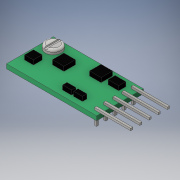
# Autodesk Inventor part: IMU
Saved by Autodesk Inventor 2016 (Build 200138000, 138)
## iProperties
Created: 2015-09-21
Part Number: IMU
Material: Generic
Document SubType Name: Modeling
Designer: lachesis
Density: 1 g/cm^3
Appearance: Default
Author: lachesis
Autodesk Inventor part; units mm, degrees
ref_plane "YZ Plane" through (0, 0, 0) normal (1, 0, 0) x (0, 1, 0)
ref_plane "XZ Plane" through (0, 0, 0) normal (0, 1, 0) x (-1, 0, 0)
ref_plane "XY Plane" through (0, 0, 0) normal (0, 0, 1) x (1, 0, 0)
sketch "Sketch1" plane through (0, 0, 0) normal (0, 1, 0) x (-1, 0, 0)
  line L0 (12.954, 6.731) -> (-12.954, 6.731)
  line L1 (-12.954, 6.731) -> (-12.954, -6.731)
  line L2 (-12.954, -6.731) -> (12.954, -6.731)
  line L3 (12.954, -6.731) -> (12.954, 6.731)
  point P0 (0, 0)
  point P1 (12.954, 0)
  point P2 (0, -6.731)
  dimension "d0" = 25.908
  dimension "d1" = 13.462
  constraints: 8 end point, 2 midpoint, 2 parallel, 1 horizontal, 1 horizontal alignment, 1 perpendicular, 1 vertical alignment
  measures "d0" distance of L1.end L2.end
  measures "d1" distance of L2.end L0.start
extrude "Extrusion1" add sketch "Sketch1" along normal blind 1.27
sketch "Sketch2" plane through (0, 1.27, 0) normal (0, 1, 0) x (1, 0, 0)
  circle A0 centre (-10.033, 3.81) radius 2.286
  line L0 (-12.954, 6.731) -> (-12.954, -6.731) projected
  line L1 (-11.303, -0.635) -> (-8.763, -0.635)
  line L2 (-8.763, -0.635) -> (-8.763, -3.175)
  line L3 (-8.763, -3.175) -> (-11.303, -3.175)
  line L4 (-11.303, -3.175) -> (-11.303, -0.635)
  line L5 (-12.954, -6.731) -> (12.954, -6.731) projected
  line L6 (-6.096, 2.921) -> (-2.794, 2.921)
  line L7 (-2.794, 2.921) -> (-2.794, -0.381)
  line L8 (-2.794, -0.381) -> (-6.096, -0.381)
  line L9 (-6.096, -0.381) -> (-6.096, 2.921)
  line L10 (12.954, 6.731) -> (-12.954, 6.731) projected
  line L11 (2.032, 5.461) -> (5.334, 5.461)
  line L12 (5.334, 5.461) -> (5.334, 2.159)
  line L13 (5.334, 2.159) -> (2.032, 2.159)
  line L14 (2.032, 2.159) -> (2.032, 5.461)
  line L15 (12.954, -6.731) -> (12.954, 6.731) projected
  line L16 (6.858, 4.699) -> (9.906, 4.699)
  line L17 (9.906, 4.699) -> (9.906, 2.667)
  line L18 (9.906, 2.667) -> (6.858, 2.667)
  line L19 (6.858, 2.667) -> (6.858, 4.699)
  line L20 (1.651, -3.937) -> (4.191, -3.937)
  line L21 (4.191, -3.937) -> (4.191, -5.207)
  line L22 (4.191, -5.207) -> (1.651, -5.207)
  line L23 (1.651, -5.207) -> (1.651, -3.937)
  line L24 (4.826, -3.937) -> (7.366, -3.937)
  line L25 (7.366, -3.937) -> (7.366, -5.207)
  line L26 (7.366, -5.207) -> (4.826, -5.207)
  line L27 (4.826, -5.207) -> (4.826, -3.937)
  point P0 (0, 0)
  point P1 (-10.033, -0.635)
  dimension "d5" = 4.572
  dimension "d9" = 2.921
  dimension "d10" = 3.81
  dimension "d11" = 2.54
  dimension "d12" = 2.54
  dimension "d13" = 3.556
  dimension "d14" = 3.302
  dimension "d15" = 3.302
  dimension "d16" = 6.858
  dimension "d17" = 3.81
  dimension "d18" = 3.302
  dimension "d19" = 3.302
  dimension "d20" = 7.62
  dimension "d21" = 1.27
  dimension "d22" = 3.048
  dimension "d23" = 2.032
  dimension "d24" = 2.032
  dimension "d25" = 3.048
  dimension "d26" = 1.524
  dimension "d27" = 2.54
  dimension "d28" = 2.54
  dimension "d29" = 1.27
  dimension "d30" = 0.635
  dimension "d31" = 5.588
  constraints: 48 end point, 12 parallel, 6 horizontal, 6 perpendicular, 2 point on line, 1 centre point, 1 midpoint, 1 vertical alignment
  measures "d5" diameter of A0
  measures "d9" distance from line of L0 A0.centre
  measures "d10" vertical distance of point (0, 0) A0.centre
  measures "d11" distance of L1.start L1.end
  measures "d12" distance of L1.end L2.end
  measures "d13" distance between parallel lines of L5 L3
  measures "d14" distance of L6.start L6.end
  measures "d15" distance of L6.end L7.end
  measures "d16" distance between parallel lines of L0 L9
  measures "d17" distance between parallel lines of L10 L6
  measures "d18" distance of L11.start L11.end
  measures "d19" distance of L11.end L12.end
  measures "d20" distance between parallel lines of L15 L12
  measures "d21" distance between parallel lines of L10 L11
  measures "d22" distance between parallel lines of L15 L17
  measures "d23" distance between parallel lines of L10 L16
  measures "d24" distance of L18.end L16.start
  measures "d25" distance of L17.end L18.end
  measures "d26" distance between parallel lines of L5 L22
  measures "d27" distance of L20.start L20.end
  measures "d28" distance of L24.start L24.end
  measures "d29" distance of L24.end L25.end
  measures "d30" distance between parallel lines of L27 L21
  measures "d31" distance between parallel lines of L15 L25
extrude "Extrusion2" add sketch "Sketch2" along normal blind 1.27 contours A0 | L1 L2 L3 L4 | L6 L7 L8 L9 | L11 L12 L13 L14 | L16 L17 L18 L19 | L20 L21 L22 L23 | L24 L25 L26 L27
fillet "Fillet1" radius 0.635 1 edges at (-12.319, 2.54, -3.81)
sketch "Sketch3" plane through (-10.033, 2.54, -3.81) normal (0, 1, 0) x (1, 0, 0)
  circle A0 centre (0, 0) radius 2.286 projected
  line L0 (-0.381, 2.254) -> (-0.381, -2.254)
  line L1 (0.381, 2.254) -> (0.381, -2.254)
  point P0 (10.033, -3.81)
  dimension "d35" = 0.762
  dimension "d36" = 0.381
  constraints: 4 end point, 4 point on circle, 1 parallel, 1 vertical
  measures "d35" distance between parallel lines of L0 L1
  measures "d36" distance from line of A0.centre L0
extrude "Extrusion3" cut sketch "Sketch3" against normal blind 0.381 contours L1 A0 L0
sketch "Sketch4" plane through (0, 1.27, 0) normal (0, 1, 0) x (1, 0, 0)
  line L0 (11.176, 5.588) -> (21.59, 5.588)
  line L1 (21.59, 5.588) -> (21.59, 4.9784)
  line L2 (21.59, 4.9784) -> (11.176, 4.9784)
  line L3 (11.176, 4.9784) -> (11.176, 5.588)
  line L4 (11.176, 2.9464) -> (21.59, 2.9464)
  line L5 (21.59, 2.9464) -> (21.59, 2.3368)
  line L6 (21.59, 2.3368) -> (11.176, 2.3368)
  line L7 (11.176, 2.3368) -> (11.176, 2.9464)
  line L8 (11.176, 0.3048) -> (21.59, 0.3048)
  line L9 (21.59, 0.3048) -> (21.59, -0.3048)
  line L10 (21.59, -0.3048) -> (11.176, -0.3048)
  line L11 (11.176, -0.3048) -> (11.176, 0.3048)
  line L12 (11.176, -2.3368) -> (21.59, -2.3368)
  line L13 (21.59, -2.3368) -> (21.59, -2.9464)
  line L14 (21.59, -2.9464) -> (11.176, -2.9464)
  line L15 (11.176, -2.9464) -> (11.176, -2.3368)
  line L16 (11.176, -4.9784) -> (21.59, -4.9784)
  line L17 (21.59, -4.9784) -> (21.59, -5.588)
  line L18 (21.59, -5.588) -> (11.176, -5.588)
  line L19 (11.176, -5.588) -> (11.176, -4.9784)
  line L20 (12.954, -6.731) -> (12.954, 6.731) projected
  line L21 (12.954, 6.731) -> (-12.954, 6.731) projected
  line L22 (11.9899, 5.588) -> (11.9899, 6.731) construction
  line L23 (11.9899, -5.588) -> (11.9899, -6.731) construction
  line L24 (-12.954, -6.731) -> (12.954, -6.731) projected
  point P0 (0, 0)
  point P1 (11.176, -2.6416)
  point P2 (11.176, 0)
  dimension "d39" = 2.032
  dimension "d40" = 2.032
  dimension "d41" = 2.032
  dimension "d42" = 2.032
  dimension "d43" = 0.6096
  dimension "d44" = 0.6096
  dimension "d45" = 0.6096
  dimension "d46" = 0.6096
  dimension "d47" = 0.6096
  dimension "d48" = 10.414
  dimension "d49" = 1.778
  dimension "d52" = 0.9641
  dimension "d53" = 0.9641
  constraints: 44 end point, 11 point on line, 10 parallel, 6 perpendicular, 5 horizontal, 2 midpoint, 1 collinear, 1 vertical, 1 vertical alignment
  measures "d39" distance between parallel lines of L4 L2
  measures "d40" distance between parallel lines of L8 L6
  measures "d41" distance between parallel lines of L12 L10
  measures "d42" distance between parallel lines of L16 L14
  measures "d43" distance of L0.end L1.end
  measures "d44" distance of L4.end L5.end
  measures "d45" distance of L8.end L9.end
  measures "d46" distance of L12.end L13.end
  measures "d47" distance of L16.end L17.end
  measures "d48" distance of L0.start L0.end
  measures "d49" distance between parallel lines of L20 L3
  measures "d52" distance between parallel lines of L22 L20
  measures "d53" distance between parallel lines of L23 L20
extrude "Extrusion4" add sketch "Sketch4" along normal blind 0.6096
ref_plane "Work Plane1" through (11.176, 1.5748, -5.588) normal (-1, 0, 0) x (0, 0, 1)
sketch "Sketch5" plane through (11.176, 1.5748, -5.588) normal (-1, 0, 0) x (0, 0, 1)
  line L0 (10.5664, -0.3048) -> (11.176, -0.3048) projected
  line L1 (10.5664, -0.3048) -> (10.5664, 0.3048) projected
  line L2 (11.176, 0.3048) -> (10.5664, 0.3048) projected
  line L3 (11.176, -0.3048) -> (11.176, 0.3048) projected
  line L4 (7.9248, -0.3048) -> (8.5344, -0.3048) projected
  line L5 (7.9248, -0.3048) -> (7.9248, 0.3048) projected
  line L6 (8.5344, 0.3048) -> (7.9248, 0.3048) projected
  line L7 (8.5344, -0.3048) -> (8.5344, 0.3048) projected
  line L8 (5.2832, -0.3048) -> (5.8928, -0.3048) projected
  line L9 (5.2832, -0.3048) -> (5.2832, 0.3048) projected
  line L10 (5.8928, 0.3048) -> (5.2832, 0.3048) projected
  line L11 (5.8928, -0.3048) -> (5.8928, 0.3048) projected
  line L12 (2.6416, -0.3048) -> (3.2512, -0.3048) projected
  line L13 (2.6416, -0.3048) -> (2.6416, 0.3048) projected
  line L14 (3.2512, 0.3048) -> (2.6416, 0.3048) projected
  line L15 (3.2512, -0.3048) -> (3.2512, 0.3048) projected
  line L16 (0, -0.3048) -> (0.6096, -0.3048) projected
  line L17 (0, -0.3048) -> (0, 0.3048) projected
  line L18 (0.6096, 0.3048) -> (0, 0.3048) projected
  line L19 (0.6096, -0.3048) -> (0.6096, 0.3048) projected
  line L20 (11.176, -0.3048) -> (10.5664, -0.3048)
  line L21 (10.5664, -0.3048) -> (10.5664, -4.1148)
  line L22 (10.5664, -4.1148) -> (11.176, -4.1148)
  line L23 (11.176, -4.1148) -> (11.176, -0.3048)
  line L24 (8.5344, -0.3048) -> (7.9248, -0.3048)
  line L25 (7.9248, -0.3048) -> (7.9248, -4.1148)
  line L26 (7.9248, -4.1148) -> (8.5344, -4.1148)
  line L27 (8.5344, -4.1148) -> (8.5344, -0.3048)
  line L28 (5.8928, -0.3048) -> (5.2832, -0.3048)
  line L29 (5.2832, -0.3048) -> (5.2832, -4.1148)
  line L30 (5.2832, -4.1148) -> (5.8928, -4.1148)
  line L31 (5.8928, -4.1148) -> (5.8928, -0.3048)
  line L32 (3.2512, -0.3048) -> (2.6416, -0.3048)
  line L33 (2.6416, -0.3048) -> (2.6416, -4.1148)
  line L34 (2.6416, -4.1148) -> (3.2512, -4.1148)
  line L35 (3.2512, -4.1148) -> (3.2512, -0.3048)
  line L36 (0.6096, -0.3048) -> (0, -0.3048)
  line L37 (0, -0.3048) -> (0, -4.1148)
  line L38 (0, -4.1148) -> (0.6096, -4.1148)
  line L39 (0.6096, -4.1148) -> (0.6096, -0.3048)
  point P0 (5.588, -1.5748)
  dimension "d56" = 3.81
  dimension "d62" = 0.6096
  dimension "d63" = 3.2512
  dimension "d64" = 5.8928
  dimension "d65" = 8.5344
  dimension "d66" = 11.176
  constraints: 40 end point, 10 parallel, 5 collinear, 5 horizontal, 5 perpendicular, 4 point on line
  measures "d56" distance of L20.end L21.end
  measures "d62" distance between parallel lines of L3 L21
  measures "d63" distance between parallel lines of L3 L25
  measures "d64" distance between parallel lines of L3 L29
  measures "d65" distance between parallel lines of L3 L33
  measures "d66" distance between parallel lines of L3 L37
extrude "Extrusion5" add sketch "Sketch5" against normal blind 0.6096 contours L0 L23 L22 L21 | L4 L27 L26 L25 | L8 L31 L30 L29 | L12 L35 L34 L33 | L16 L39 L38 L37
equation "\"d12\" = d11"
equation "\"d15\" = d14"
equation "\"d18\" = d14"
equation "\"d19\" = d18"
equation "\"d28\" = d27"
equation "\"d36\" = 0.5 * d35"
equation "\"d40\" = d39"
equation "\"d41\" = d39"
equation "\"d42\" = d39"
equation "\"d44\" = d43"
equation "\"d45\" = d44"
equation "\"d46\" = d45"
equation "\"d47\" = d46"
body "Solid1"
